Autodesk Inventor part; units mm, degrees
(part 2 of 2)
sketch "Sketch26" plane through (0, 0, 0) normal (0, -1, 0) x (1, 0, 0)
  circle A0 centre (0, 0) radius 23.8125 construction
  spline S0 degree 2 poles (-24.8851, 3.9966) (-24.5644, 3.9692) (-24.1006, 3.6837) (-23.9576, 3.4678) knots 0 0 0 1 2 2 2
  spline S1 degree 2 poles (-23.9576, 3.4678) (-23.7867, 3.2073) (-23.6758, 2.6148) (-23.7143, 2.1651) knots 0 0 0 1 2 2 2
  line L0 (-23.7143, 2.1651) -> (-23.8613, 0.4463)
  line L1 (-23.8613, 0.4463) -> (-28.1636, 0.8142)
  line L2 (-28.1636, 0.8142) -> (-28.0338, 2.3308)
  spline S2 degree 2 poles (-28.0338, 2.3308) (-27.9933, 2.805) (-27.8783, 3.2868) (-27.7451, 3.4897) knots 0 0 0 1 2 2 2
  spline S3 degree 2 poles (-27.7451, 3.4897) (-27.6031, 3.7128) (-27.1653, 3.9037) (-26.8934, 3.8804) knots 0 0 0 1 2 2 2
  spline S4 degree 2 poles (-26.8934, 3.8804) (-26.5796, 3.8536) (-26.1149, 3.4977) (-26.0237, 3.209) knots 0 0 0 1 2 2 2
  line L3 (-26.0237, 3.209) -> (-26.0027, 3.2072)
  spline S5 degree 2 poles (-26.0027, 3.2072) (-25.8848, 3.601) (-25.3244, 4.0342) (-24.8851, 3.9966) knots 0 0 0 1 2 2 2
  spline S6 degree 2 poles (-24.998, 2.8825) (-25.2002, 2.8997) (-25.4405, 2.7588) (-25.5135, 2.6034) knots 0 0 0 1 2 2 2
  spline S7 degree 2 poles (-25.5135, 2.6034) (-25.5602, 2.5091) (-25.5967, 2.1645) (-25.6212, 1.8786) knots 0 0 0 1 2 2 2
  line L4 (-25.6212, 1.8786) -> (-25.6382, 1.6799)
  line L5 (-25.6382, 1.6799) -> (-24.5539, 1.5872)
  line L6 (-24.5539, 1.5872) -> (-24.5488, 1.6465)
  spline S8 degree 2 poles (-24.5488, 1.6465) (-24.513, 2.0648) (-24.4961, 2.3865) (-24.555, 2.5601) knots 0 0 0 1 2 2 2
  spline S9 degree 2 poles (-24.555, 2.5601) (-24.6087, 2.7122) (-24.8411, 2.869) (-24.998, 2.8825) knots 0 0 0 1 2 2 2
  spline S10 degree 2 poles (-26.7746, 2.764) (-26.8792, 2.7729) (-27.1081, 2.6836) (-27.1665, 2.5762) knots 0 0 0 1 2 2 2
  spline S11 degree 2 poles (-27.1665, 2.5762) (-27.2242, 2.4758) (-27.2563, 2.1835) (-27.281, 1.8942) knots 0 0 0 1 2 2 2
  line L7 (-27.281, 1.8942) -> (-27.2873, 1.821)
  line L8 (-27.2873, 1.821) -> (-26.3738, 1.7428)
  line L9 (-26.3738, 1.7428) -> (-26.3622, 1.8788)
  spline S12 degree 2 poles (-26.3622, 1.8788) (-26.3386, 2.1542) (-26.33, 2.3783) (-26.3756, 2.5016) knots 0 0 0 1 2 2 2
  spline S13 degree 2 poles (-26.3756, 2.5016) (-26.4274, 2.6359) (-26.6317, 2.7518) (-26.7746, 2.764) knots 0 0 0 1 2 2 2
  spline S14 degree 2 poles (-24.2532, 7.8601) (-23.4729, 7.663) (-22.7924, 6.5852) (-22.9886, 5.8083) knots 0 0 0 1 2 2 2
  spline S15 degree 2 poles (-22.9886, 5.8083) (-23.184, 5.0348) (-24.2964, 4.4027) (-25.0768, 4.5998) knots 0 0 0 1 2 2 2
  spline S16 degree 2 poles (-25.0768, 4.5998) (-25.8638, 4.7986) (-26.5393, 5.8823) (-26.3439, 6.6558) knots 0 0 0 1 2 2 2
  spline S17 degree 2 poles (-26.3439, 6.6558) (-26.1486, 7.4293) (-25.0369, 8.0581) (-24.2532, 7.8601) knots 0 0 0 1 2 2 2
  spline S18 degree 2 poles (-24.501, 6.8508) (-24.7826, 6.9219) (-25.1823, 6.9254) (-25.3148, 6.8723) knots 0 0 0 1 2 2 2
  spline S19 degree 2 poles (-25.3148, 6.8723) (-25.4558, 6.8141) (-25.6031, 6.6167) (-25.6383, 6.4776) knots 0 0 0 1 2 2 2
  spline S20 degree 2 poles (-25.6383, 6.4776) (-25.6725, 6.3419) (-25.6451, 6.1076) (-25.552, 5.9902) knots 0 0 0 1 2 2 2
  spline S21 degree 2 poles (-25.552, 5.9902) (-25.4649, 5.878) (-25.1072, 5.6794) (-24.8155, 5.6057) knots 0 0 0 1 2 2 2
  spline S22 degree 2 poles (-24.8155, 5.6057) (-24.5271, 5.5328) (-24.1469, 5.5379) (-24.0186, 5.5885) knots 0 0 0 1 2 2 2
  spline S23 degree 2 poles (-24.0186, 5.5885) (-23.8903, 5.6391) (-23.7286, 5.8509) (-23.6926, 5.9933) knots 0 0 0 1 2 2 2
  spline S24 degree 2 poles (-23.6926, 5.9933) (-23.6626, 6.1121) (-23.7027, 6.3821) (-23.7856, 6.4824) knots 0 0 0 1 2 2 2
  spline S25 degree 2 poles (-23.7856, 6.4824) (-23.8829, 6.5972) (-24.2024, 6.7754) (-24.501, 6.8508) knots 0 0 0 1 2 2 2
  spline S26 degree 2 poles (-21.9439, 9.0922) (-22.1712, 8.5161) (-22.8546, 8.1763) (-23.3949, 8.3896) knots 0 0 0 1 2 2 2
  line L10 (-23.3949, 8.3896) -> (-24.8107, 8.9484)
  line L11 (-24.8107, 8.9484) -> (-24.9533, 8.5872)
  line L12 (-24.9533, 8.5872) -> (-25.6108, 8.8467)
  line L13 (-25.6108, 8.8467) -> (-25.4682, 9.208)
  line L14 (-25.4682, 9.208) -> (-26.334, 9.5497)
  line L15 (-26.334, 9.5497) -> (-25.9614, 10.4936)
  line L16 (-25.9614, 10.4936) -> (-25.0956, 10.1519)
  line L17 (-25.0956, 10.1519) -> (-24.7359, 11.0632)
  line L18 (-24.7359, 11.0632) -> (-24.0784, 10.8037)
  line L19 (-24.0784, 10.8037) -> (-24.4382, 9.8923)
  line L20 (-24.4382, 9.8923) -> (-23.3608, 9.4671)
  spline S27 degree 2 poles (-23.3608, 9.4671) (-23.2013, 9.4042) (-22.9611, 9.3169) (-22.8513, 9.3187) knots 0 0 0 1 2 2 2
  spline S28 degree 2 poles (-22.8513, 9.3187) (-22.7415, 9.3205) (-22.5551, 9.4688) (-22.4831, 9.6511) knots 0 0 0 1 2 2 2
  spline S29 degree 2 poles (-22.4831, 9.6511) (-22.4523, 9.7292) (-22.421, 9.999) (-22.4278, 10.0581) knots 0 0 0 1 2 2 2
  line L21 (-22.4278, 10.0581) -> (-22.3957, 10.1395)
  line L22 (-22.3957, 10.1395) -> (-21.7317, 9.8774)
  spline S30 degree 2 poles (-21.7317, 9.8774) (-21.753, 9.709) (-21.8436, 9.346) (-21.9439, 9.0922) knots 0 0 0 1 2 2 2
  spline S31 degree 2 poles (-20.887, 11.3108) (-21.1727, 10.7612) (-21.8875, 10.4939) (-22.4028, 10.7619) knots 0 0 0 1 2 2 2
  line L23 (-22.4028, 10.7619) -> (-23.7534, 11.464)
  line L24 (-23.7534, 11.464) -> (-23.9325, 11.1194)
  line L25 (-23.9325, 11.1194) -> (-24.5597, 11.4455)
  line L26 (-24.5597, 11.4455) -> (-24.3805, 11.7901)
  line L27 (-24.3805, 11.7901) -> (-25.2064, 12.2194)
  line L28 (-25.2064, 12.2194) -> (-24.7383, 13.1198)
  line L29 (-24.7383, 13.1198) -> (-23.9124, 12.6904)
  line L30 (-23.9124, 12.6904) -> (-23.4605, 13.5597)
  line L31 (-23.4605, 13.5597) -> (-22.8333, 13.2337)
  line L32 (-22.8333, 13.2337) -> (-23.2853, 12.3644)
  line L33 (-23.2853, 12.3644) -> (-22.2576, 11.8301)
  spline S32 degree 2 poles (-22.2576, 11.8301) (-22.1055, 11.751) (-21.8756, 11.6394) (-21.7662, 11.6298) knots 0 0 0 1 2 2 2
  spline S33 degree 2 poles (-21.7662, 11.6298) (-21.6568, 11.6203) (-21.456, 11.7486) (-21.3656, 11.9224) knots 0 0 0 1 2 2 2
  spline S34 degree 2 poles (-21.3656, 11.9224) (-21.3269, 11.9969) (-21.2679, 12.2621) (-21.2686, 12.3216) knots 0 0 0 1 2 2 2
  line L34 (-21.2686, 12.3216) -> (-21.2282, 12.3992)
  line L35 (-21.2282, 12.3992) -> (-20.5949, 12.0699)
  spline S35 degree 2 poles (-20.5949, 12.0699) (-20.6335, 11.9046) (-20.7611, 11.5529) (-20.887, 11.3108) knots 0 0 0 1 2 2 2
  spline S36 degree 2 poles (-19.9207, 15.9113) (-19.2601, 15.4515) (-19.0035, 14.203) (-19.4612, 13.5452) knots 0 0 0 1 2 2 2
  spline S37 degree 2 poles (-19.4612, 13.5452) (-19.9169, 12.8904) (-21.1809, 12.6914) (-21.8415, 13.1511) knots 0 0 0 1 2 2 2
  spline S38 degree 2 poles (-21.8415, 13.1511) (-22.5078, 13.6148) (-22.7575, 14.8671) (-22.3018, 15.522) knots 0 0 0 1 2 2 2
  spline S39 degree 2 poles (-22.3018, 15.522) (-21.8461, 16.1769) (-20.5841, 16.373) (-19.9207, 15.9113) knots 0 0 0 1 2 2 2
  spline S40 degree 2 poles (-20.5086, 15.0542) (-20.7469, 15.2201) (-21.1197, 15.3644) (-21.2625, 15.3615) knots 0 0 0 1 2 2 2
  spline S41 degree 2 poles (-21.2625, 15.3615) (-21.415, 15.3567) (-21.6224, 15.224) (-21.7044, 15.1063) knots 0 0 0 1 2 2 2
  spline S42 degree 2 poles (-21.7044, 15.1063) (-21.7843, 14.9914) (-21.8413, 14.7625) (-21.7956, 14.6198) knots 0 0 0 1 2 2 2
  spline S43 degree 2 poles (-21.7956, 14.6198) (-21.7537, 14.4841) (-21.4891, 14.172) (-21.2421, 14.0001) knots 0 0 0 1 2 2 2
  spline S44 degree 2 poles (-21.2421, 14.0001) (-20.998, 13.8302) (-20.6404, 13.7008) (-20.5025, 13.7029) knots 0 0 0 1 2 2 2
  spline S45 degree 2 poles (-20.5025, 13.7029) (-20.3647, 13.705) (-20.1386, 13.8461) (-20.0546, 13.9667) knots 0 0 0 1 2 2 2
  spline S46 degree 2 poles (-20.0546, 13.9667) (-19.9847, 14.0672) (-19.9269, 14.334) (-19.9691, 14.4572) knots 0 0 0 1 2 2 2
  spline S47 degree 2 poles (-19.9691, 14.4572) (-20.0197, 14.5989) (-20.2558, 14.8783) (-20.5086, 15.0542) knots 0 0 0 1 2 2 2
  line L36 (-15.498, 18.1366) -> (-16.628, 19.3073)
  spline S48 degree 2 poles (-16.628, 19.3073) (-16.7957, 19.481) (-17.0367, 19.7055) (-17.1399, 19.7519) knots 0 0 0 1 2 2 2
  spline S49 degree 2 poles (-17.1399, 19.7519) (-17.2455, 19.7958) (-17.442, 19.7374) (-17.5604, 19.6232) knots 0 0 0 1 2 2 2
  spline S50 degree 2 poles (-17.5604, 19.6232) (-17.6434, 19.543) (-17.7341, 19.3145) (-17.7641, 19.1541) knots 0 0 0 1 2 2 2
  line L37 (-17.7641, 19.1541) -> (-16.1627, 17.495)
  line L38 (-16.1627, 17.495) -> (-16.8978, 16.7854)
  line L39 (-16.8978, 16.7854) -> (-18.0278, 17.9561)
  spline S51 degree 2 poles (-18.0278, 17.9561) (-18.1931, 18.1273) (-18.4391, 18.3519) (-18.5422, 18.3983) knots 0 0 0 1 2 2 2
  spline S52 degree 2 poles (-18.5422, 18.3983) (-18.6478, 18.4422) (-18.8444, 18.3838) (-18.9627, 18.2696) knots 0 0 0 1 2 2 2
  spline S53 degree 2 poles (-18.9627, 18.2696) (-19.0508, 18.1845) (-19.1443, 17.9338) (-19.169, 17.7981) knots 0 0 0 1 2 2 2
  line L40 (-19.169, 17.7981) -> (-17.5675, 16.139)
  line L41 (-17.5675, 16.139) -> (-18.2976, 15.4342)
  line L42 (-18.2976, 15.4342) -> (-20.5601, 17.7781)
  line L43 (-20.5601, 17.7781) -> (-19.83, 18.4829)
  line L44 (-19.83, 18.4829) -> (-19.5797, 18.2236)
  spline S54 degree 2 poles (-19.5797, 18.2236) (-19.5468, 18.5472) (-19.3923, 19.027) (-19.1934, 19.219) knots 0 0 0 1 2 2 2
  spline S55 degree 2 poles (-19.1934, 19.219) (-18.9794, 19.4256) (-18.4552, 19.5376) (-18.1728, 19.4163) knots 0 0 0 1 2 2 2
  spline S56 degree 2 poles (-18.1728, 19.4163) (-18.1534, 19.8143) (-17.9849, 20.3855) (-17.7936, 20.5702) knots 0 0 0 1 2 2 2
  spline S57 degree 2 poles (-17.7936, 20.5702) (-17.6299, 20.7281) (-17.271, 20.8752) (-17.0808, 20.8545) knots 0 0 0 1 2 2 2
  spline S58 degree 2 poles (-17.0808, 20.8545) (-16.8732, 20.836) (-16.4761, 20.6211) (-16.2355, 20.3719) knots 0 0 0 1 2 2 2
  line L45 (-16.2355, 20.3719) -> (-14.7628, 18.8462)
  line L46 (-14.7628, 18.8462) -> (-15.498, 18.1366)
  line L47 (-9.4111, 21.9496) -> (-10.3726, 21.4473)
  line L48 (-10.3726, 21.4473) -> (-11.2588, 23.1438)
  line L49 (-11.2588, 23.1438) -> (-12.5646, 22.4617)
  line L50 (-12.5646, 22.4617) -> (-11.6783, 20.7652)
  line L51 (-11.6783, 20.7652) -> (-12.6398, 20.263)
  line L52 (-12.6398, 20.263) -> (-14.6391, 24.0902)
  line L53 (-14.6391, 24.0902) -> (-13.6776, 24.5925)
  line L54 (-13.6776, 24.5925) -> (-12.9453, 23.1906)
  line L55 (-12.9453, 23.1906) -> (-11.6396, 23.8727)
  line L56 (-11.6396, 23.8727) -> (-12.3719, 25.2746)
  line L57 (-12.3719, 25.2746) -> (-11.4104, 25.7768)
  line L58 (-11.4104, 25.7768) -> (-9.4111, 21.9496)
  spline S59 degree 2 poles (-7.0133, 22.6666) (-7.8923, 22.3827) (-9.0991, 22.9195) (-9.3497, 23.6954) knots 0 0 0 1 2 2 2
  spline S60 degree 2 poles (-9.3497, 23.6954) (-9.5949, 24.4546) (-9.0151, 25.6421) (-8.2293, 25.8959) knots 0 0 0 1 2 2 2
  spline S61 degree 2 poles (-8.2293, 25.8959) (-7.52, 26.125) (-6.5523, 25.5882) (-6.3221, 24.8756) knots 0 0 0 1 2 2 2
  line L59 (-6.3221, 24.8756) -> (-6.2092, 24.526)
  line L60 (-6.2092, 24.526) -> (-8.3303, 23.8408)
  spline S62 degree 2 poles (-8.3303, 23.8408) (-8.247, 23.6287) (-7.998, 23.3929) (-7.8435, 23.3472) knots 0 0 0 1 2 2 2
  spline S63 degree 2 poles (-7.8435, 23.3472) (-7.6924, 23.3004) (-7.3357, 23.3347) (-7.1393, 23.3982) knots 0 0 0 1 2 2 2
  spline S64 degree 2 poles (-7.1393, 23.3982) (-6.9728, 23.452) (-6.6701, 23.6306) (-6.554, 23.738) knots 0 0 0 1 2 2 2
  spline S65 degree 2 poles (-6.554, 23.738) (-6.4503, 23.8267) (-6.2903, 24.0144) (-6.2421, 24.0814) knots 0 0 0 1 2 2 2
  line L61 (-6.2421, 24.0814) -> (-6.1389, 24.1148)
  line L62 (-6.1389, 24.1148) -> (-5.8807, 23.3156)
  spline S66 degree 2 poles (-5.8807, 23.3156) (-5.9855, 23.2303) (-6.1529, 23.088) (-6.3131, 22.9921) knots 0 0 0 1 2 2 2
  spline S67 degree 2 poles (-6.3131, 22.9921) (-6.4556, 22.8983) (-6.7735, 22.7441) (-7.0133, 22.6666) knots 0 0 0 1 2 2 2
  spline S68 degree 2 poles (-7.3498, 24.8011) (-7.4554, 25.1053) (-7.8294, 25.3411) (-8.1058, 25.2518) knots 0 0 0 1 2 2 2
  spline S69 degree 2 poles (-8.1058, 25.2518) (-8.3888, 25.1604) (-8.5988, 24.7175) (-8.5218, 24.4224) knots 0 0 0 1 2 2 2
  line L63 (-8.5218, 24.4224) -> (-7.3498, 24.8011)
  line L64 (-2.0894, 23.7885) -> (-3.2634, 23.5956)
  line L65 (-3.2634, 23.5956) -> (-4.026, 24.4171)
  line L66 (-4.026, 24.4171) -> (-4.5029, 23.3919)
  line L67 (-4.5029, 23.3919) -> (-5.6528, 23.203)
  line L68 (-5.6528, 23.203) -> (-4.7328, 25.0066)
  line L69 (-4.7328, 25.0066) -> (-6.1602, 26.4211)
  line L70 (-6.1602, 26.4211) -> (-4.9862, 26.6139)
  line L71 (-4.9862, 26.6139) -> (-4.2368, 25.808)
  line L72 (-4.2368, 25.808) -> (-3.7812, 26.8119)
  line L73 (-3.7812, 26.8119) -> (-2.6314, 27.0009)
  line L74 (-2.6314, 27.0009) -> (-3.5352, 25.2282)
  line L75 (-3.5352, 25.2282) -> (-2.0894, 23.7885)
  line L76 (-0.4845, 23.8131) -> (-1.5088, 23.7701)
  line L77 (-1.5088, 23.7701) -> (-1.5566, 24.9099)
  line L78 (-1.5566, 24.9099) -> (-0.5323, 24.9529)
  line L79 (-0.5323, 24.9529) -> (-0.4845, 23.8131)
  line L80 (-0.5732, 25.9283) -> (-1.5976, 25.8853)
  line L81 (-1.5976, 25.8853) -> (-1.6454, 27.025)
  line L82 (-1.6454, 27.025) -> (-0.621, 27.068)
  line L83 (-0.621, 27.068) -> (-0.5732, 25.9283)
  spline S70 degree 2 poles (5.6673, 25.4002) (5.5806, 24.8471) (5.2742, 24.045) (5.0332, 23.7959) knots 0 0 0 1 2 2 2
  spline S71 degree 2 poles (5.0332, 23.7959) (4.7963, 23.5497) (4.1261, 23.3644) (3.6767, 23.4349) knots 0 0 0 1 2 2 2
  spline S72 degree 2 poles (3.6767, 23.4349) (3.2239, 23.5059) (2.6461, 23.8869) (2.4935, 24.2013) knots 0 0 0 1 2 2 2
  spline S73 degree 2 poles (2.4935, 24.2013) (2.3403, 24.5122) (2.2931, 25.3626) (2.3798, 25.9157) knots 0 0 0 1 2 2 2
  spline S74 degree 2 poles (2.3798, 25.9157) (2.4687, 26.4826) (2.7708, 27.257) (3.0168, 27.5159) knots 0 0 0 1 2 2 2
  spline S75 degree 2 poles (3.0168, 27.5159) (3.2618, 27.768) (3.9378, 27.9453) (4.3733, 27.877) knots 0 0 0 1 2 2 2
  spline S76 degree 2 poles (4.3733, 27.877) (4.8331, 27.8049) (5.4029, 27.418) (5.555, 27.1002) knots 0 0 0 1 2 2 2
  spline S77 degree 2 poles (5.555, 27.1002) (5.7046, 26.7898) (5.7514, 25.936) (5.6673, 25.4002) knots 0 0 0 1 2 2 2
  spline S78 degree 2 poles (4.5922, 25.5688) (4.7164, 26.3604) (4.5574, 27.0406) (4.2497, 27.0888) knots 0 0 0 1 2 2 2
  spline S79 degree 2 poles (4.2497, 27.0888) (3.9421, 27.1371) (3.579, 26.5388) (3.4544, 25.7437) knots 0 0 0 1 2 2 2
  spline S80 degree 2 poles (3.4544, 25.7437) (3.3318, 24.9624) (3.4927, 24.2713) (3.8003, 24.223) knots 0 0 0 1 2 2 2
  spline S81 degree 2 poles (3.8003, 24.223) (4.1045, 24.1753) (4.4692, 24.784) (4.5922, 25.5688) knots 0 0 0 1 2 2 2
  line L84 (6.9289, 22.7878) -> (5.9419, 23.065)
  line L85 (5.9419, 23.065) -> (6.2502, 24.1633)
  line L86 (6.2502, 24.1633) -> (7.2373, 23.8861)
  line L87 (7.2373, 23.8861) -> (6.9289, 22.7878)
  spline S82 degree 2 poles (11.1529, 22.7394) (11.0232, 22.4257) (10.5906, 21.9835) (10.3015, 21.8796) knots 0 0 0 1 2 2 2
  spline S83 degree 2 poles (10.3015, 21.8796) (10.0125, 21.7757) (9.35, 21.8034) (8.9296, 21.9771) knots 0 0 0 1 2 2 2
  spline S84 degree 2 poles (8.9296, 21.9771) (8.4846, 22.1648) (7.9045, 22.5749) (7.733, 22.7556) knots 0 0 0 1 2 2 2
  line L88 (7.733, 22.7556) -> (8.0925, 23.6255)
  line L89 (8.0925, 23.6255) -> (8.1831, 23.5881)
  spline S85 degree 2 poles (8.1831, 23.5881) (8.2433, 23.514) (8.3854, 23.3265) (8.5134, 23.2055) knots 0 0 0 1 2 2 2
  spline S86 degree 2 poles (8.5134, 23.2055) (8.6329, 23.0917) (8.8965, 22.8957) (9.0744, 22.8222) knots 0 0 0 1 2 2 2
  spline S87 degree 2 poles (9.0744, 22.8222) (9.2296, 22.758) (9.6239, 22.686) (9.7766, 22.744) knots 0 0 0 1 2 2 2
  spline S88 degree 2 poles (9.7766, 22.744) (9.8908, 22.7914) (10.0629, 22.9513) (10.1311, 23.1162) knots 0 0 0 1 2 2 2
  spline S89 degree 2 poles (10.1311, 23.1162) (10.1899, 23.2585) (10.1563, 23.5071) (10.0879, 23.6073) knots 0 0 0 1 2 2 2
  spline S90 degree 2 poles (10.0879, 23.6073) (9.9895, 23.754) (9.6229, 23.9661) (9.4838, 24.0236) knots 0 0 0 1 2 2 2
  spline S91 degree 2 poles (9.4838, 24.0236) (9.2639, 24.1145) (8.8173, 24.2157) (8.6493, 24.2398) knots 0 0 0 1 2 2 2
  line L90 (8.6493, 24.2398) -> (8.562, 24.2758)
  line L91 (8.562, 24.2758) -> (9.4882, 26.5169)
  line L92 (9.4882, 26.5169) -> (12.1335, 25.4236)
  line L93 (12.1335, 25.4236) -> (11.8221, 24.6701)
  line L94 (11.8221, 24.6701) -> (10.1243, 25.3718)
  line L95 (10.1243, 25.3718) -> (9.8503, 24.7089)
  spline S92 degree 2 poles (9.8503, 24.7089) (9.9338, 24.6819) (10.1597, 24.5962) (10.2211, 24.5708) knots 0 0 0 1 2 2 2
  spline S93 degree 2 poles (10.2211, 24.5708) (10.5089, 24.4518) (10.9459, 24.1349) (11.0872, 23.9364) knots 0 0 0 1 2 2 2
  spline S94 degree 2 poles (11.0872, 23.9364) (11.2521, 23.6941) (11.2999, 23.0951) (11.1529, 22.7394) knots 0 0 0 1 2 2 2
  line L96 (14.4928, 20.2273) -> (13.9948, 20.533)
  line L97 (13.9948, 20.533) -> (13.4622, 19.6651)
  line L98 (13.4622, 19.6651) -> (12.5705, 20.2123)
  line L99 (12.5705, 20.2123) -> (13.1031, 21.0802)
  line L100 (13.1031, 21.0802) -> (11.4807, 22.0759)
  line L101 (11.4807, 22.0759) -> (11.9016, 22.7618)
  line L102 (11.9016, 22.7618) -> (14.8047, 23.9198)
  line L103 (14.8047, 23.9198) -> (15.7262, 23.3543)
  line L104 (15.7262, 23.3543) -> (14.4011, 21.1951)
  line L105 (14.4011, 21.1951) -> (14.8992, 20.8894)
  line L106 (14.8992, 20.8894) -> (14.4928, 20.2273)
  line L107 (13.5094, 21.7423) -> (14.2781, 22.9949)
  line L108 (14.2781, 22.9949) -> (12.5759, 22.3152)
  line L109 (12.5759, 22.3152) -> (13.5094, 21.7423)
  spline S95 degree 2 poles (18.1713, 18.6304) (17.8068, 18.2054) (17.1246, 17.6842) (16.7886, 17.5989) knots 0 0 0 1 2 2 2
  spline S96 degree 2 poles (16.7886, 17.5989) (16.4577, 17.514) (15.7901, 17.7085) (15.4448, 18.0047) knots 0 0 0 1 2 2 2
  spline S97 degree 2 poles (15.4448, 18.0047) (15.0969, 18.3031) (14.8056, 18.9309) (14.841, 19.2786) knots 0 0 0 1 2 2 2
  spline S98 degree 2 poles (14.841, 19.2786) (14.8741, 19.6236) (15.2809, 20.3719) (15.6454, 20.7969) knots 0 0 0 1 2 2 2
  spline S99 degree 2 poles (15.6454, 20.7969) (16.019, 21.2325) (16.6829, 21.7325) (17.0283, 21.8235) knots 0 0 0 1 2 2 2
  spline S100 degree 2 poles (17.0283, 21.8235) (17.3692, 21.9091) (18.0375, 21.7047) (18.3722, 21.4177) knots 0 0 0 1 2 2 2
  spline S101 degree 2 poles (18.3722, 21.4177) (18.7254, 21.1147) (19.0068, 20.4861) (18.9692, 20.1358) knots 0 0 0 1 2 2 2
  spline S102 degree 2 poles (18.9692, 20.1358) (18.9334, 19.7931) (18.5244, 19.0421) (18.1713, 18.6304) knots 0 0 0 1 2 2 2
  spline S103 degree 2 poles (17.3452, 19.3389) (17.8669, 19.9471) (18.0892, 20.6094) (17.8528, 20.8121) knots 0 0 0 1 2 2 2
  spline S104 degree 2 poles (17.8528, 20.8121) (17.6164, 21.0149) (16.9931, 20.6966) (16.4691, 20.0857) knots 0 0 0 1 2 2 2
  spline S105 degree 2 poles (16.4691, 20.0857) (15.9543, 19.4855) (15.7278, 18.813) (15.9642, 18.6102) knots 0 0 0 1 2 2 2
  spline S106 degree 2 poles (15.9642, 18.6102) (16.198, 18.4098) (16.8281, 18.736) (17.3452, 19.3389) knots 0 0 0 1 2 2 2
  line L110 (19.6677, 13.4747) -> (18.2626, 15.3252)
  line L111 (18.2626, 15.3252) -> (18.8618, 15.7801)
  line L112 (18.8618, 15.7801) -> (19.2363, 15.2869)
  line L113 (19.2363, 15.2869) -> (21.477, 16.9881)
  line L114 (21.477, 16.9881) -> (21.1025, 17.4814)
  line L115 (21.1025, 17.4814) -> (21.7016, 17.9364)
  line L116 (21.7016, 17.9364) -> (23.1067, 16.0859)
  line L117 (23.1067, 16.0859) -> (22.5075, 15.6309)
  line L118 (22.5075, 15.6309) -> (22.133, 16.1242)
  line L119 (22.133, 16.1242) -> (19.8923, 14.4229)
  line L120 (19.8923, 14.4229) -> (20.2669, 13.9296)
  line L121 (20.2669, 13.9296) -> (19.6677, 13.4747)
  spline S107 degree 2 poles (23.8248, 10.5322) (23.2921, 10.2446) (22.2036, 10.2573) (21.7876, 10.49) knots 0 0 0 1 2 2 2
  spline S108 degree 2 poles (21.7876, 10.49) (21.4371, 10.6825) (20.9506, 11.3185) (20.7394, 11.7096) knots 0 0 0 1 2 2 2
  line L122 (20.7394, 11.7096) -> (20.0977, 12.8981)
  line L123 (20.0977, 12.8981) -> (23.8972, 14.9496)
  line L124 (23.8972, 14.9496) -> (24.5323, 13.7735)
  spline S109 degree 2 poles (24.5323, 13.7735) (24.7484, 13.3732) (25.0242, 12.6194) (24.9934, 12.2051) knots 0 0 0 1 2 2 2
  spline S110 degree 2 poles (24.9934, 12.2051) (24.9544, 11.7029) (24.3759, 10.8298) (23.8248, 10.5322) knots 0 0 0 1 2 2 2
  spline S111 degree 2 poles (23.3023, 11.5147) (23.6779, 11.7175) (24.074, 12.2654) (24.0819, 12.6117) knots 0 0 0 1 2 2 2
  spline S112 degree 2 poles (24.0819, 12.6117) (24.0818, 12.8622) (23.874, 13.2987) (23.7144, 13.5943) knots 0 0 0 1 2 2 2
  line L125 (23.7144, 13.5943) -> (23.7044, 13.6128)
  line L126 (23.7044, 13.6128) -> (21.3243, 12.3276)
  line L127 (21.3243, 12.3276) -> (21.3343, 12.3091)
  spline S113 degree 2 poles (21.3343, 12.3091) (21.5072, 11.9889) (21.7665, 11.5603) (22.0008, 11.4283) knots 0 0 0 1 2 2 2
  spline S114 degree 2 poles (22.0008, 11.4283) (22.2749, 11.2741) (22.9266, 11.3118) (23.3023, 11.5147) knots 0 0 0 1 2 2 2
  line L128 (24.4852, 8.5487) -> (24.1281, 9.5098)
  line L129 (24.1281, 9.5098) -> (25.1974, 9.9071)
  line L130 (25.1974, 9.9071) -> (25.5545, 8.946)
  line L131 (25.5545, 8.946) -> (24.4852, 8.5487)
  line L132 (22.5007, 7.8114) -> (22.1436, 8.7725)
  line L133 (22.1436, 8.7725) -> (23.2129, 9.1698)
  line L134 (23.2129, 9.1698) -> (23.57, 8.2087)
  line L135 (23.57, 8.2087) -> (22.5007, 7.8114)
  line L136 (23.7556, 2.2444) -> (23.3062, 5.0606)
  line L137 (23.3062, 5.0606) -> (24.0491, 5.1792)
  line L138 (24.0491, 5.1792) -> (24.1925, 4.2807)
  line L139 (24.1925, 4.2807) -> (26.4489, 4.6408)
  line L140 (26.4489, 4.6408) -> (26.3056, 5.5393)
  line L141 (26.3056, 5.5393) -> (27.0001, 5.6501)
  spline S115 degree 2 poles (27.0001, 5.6501) (27.0315, 5.4531) (27.1457, 5.0709) (27.2197, 4.9623) knots 0 0 0 1 2 2 2
  spline S116 degree 2 poles (27.2197, 4.9623) (27.3103, 4.8386) (27.5661, 4.7235) (27.7411, 4.7372) knots 0 0 0 1 2 2 2
  line L142 (27.7411, 4.7372) -> (27.89, 3.8042)
  line L143 (27.89, 3.8042) -> (24.3585, 3.2406)
  line L144 (24.3585, 3.2406) -> (24.4986, 2.363)
  line L145 (24.4986, 2.363) -> (23.7556, 2.2444)
  line L146 (23.8138, 0.4435) -> (23.7728, 1.468)
  line L147 (23.7728, 1.468) -> (24.9126, 1.5137)
  line L148 (24.9126, 1.5137) -> (24.9537, 0.4892)
  line L149 (24.9537, 0.4892) -> (23.8138, 0.4435)
  spline S117 degree 2 poles (25.0716, -3.5891) (24.7332, -3.5626) (24.1791, -3.2876) (23.991, -3.0447) knots 0 0 0 1 2 2 2
  spline S118 degree 2 poles (23.991, -3.0447) (23.8029, -2.8019) (23.6248, -2.1631) (23.6603, -1.7096) knots 0 0 0 1 2 2 2
  spline S119 degree 2 poles (23.6603, -1.7096) (23.7014, -1.2285) (23.9125, -0.5501) (24.0314, -0.3312) knots 0 0 0 1 2 2 2
  line L150 (24.0314, -0.3312) -> (24.9698, -0.4047)
  line L151 (24.9698, -0.4047) -> (24.9621, -0.5023)
  spline S120 degree 2 poles (24.9621, -0.5023) (24.9102, -0.5825) (24.7758, -0.7756) (24.7002, -0.9346) knots 0 0 0 1 2 2 2
  spline S121 degree 2 poles (24.7002, -0.9346) (24.6289, -1.0835) (24.5238, -1.3946) (24.5088, -1.5865) knots 0 0 0 1 2 2 2
  spline S122 degree 2 poles (24.5088, -1.5865) (24.4957, -1.754) (24.5488, -2.1512) (24.6511, -2.2786) knots 0 0 0 1 2 2 2
  spline S123 degree 2 poles (24.6511, -2.2786) (24.7315, -2.3726) (24.9367, -2.4869) (25.1146, -2.5009) knots 0 0 0 1 2 2 2
  spline S124 degree 2 poles (25.1146, -2.5009) (25.2681, -2.5129) (25.4942, -2.4042) (25.5684, -2.3082) knots 0 0 0 1 2 2 2
  spline S125 degree 2 poles (25.5684, -2.3082) (25.6776, -2.1694) (25.7661, -1.7551) (25.7779, -1.6051) knots 0 0 0 1 2 2 2
  spline S126 degree 2 poles (25.7779, -1.6051) (25.7964, -1.3679) (25.7549, -0.9119) (25.7259, -0.7446) knots 0 0 0 1 2 2 2
  line L152 (25.7259, -0.7446) -> (25.7333, -0.6504)
  line L153 (25.7333, -0.6504) -> (28.1508, -0.8397)
  line L154 (28.1508, -0.8397) -> (27.9275, -3.6933)
  line L155 (27.9275, -3.6933) -> (27.1146, -3.6296)
  line L156 (27.1146, -3.6296) -> (27.258, -1.7982)
  line L157 (27.258, -1.7982) -> (26.5428, -1.7422)
  spline S127 degree 2 poles (26.5428, -1.7422) (26.543, -1.83) (26.5311, -2.0712) (26.5259, -2.1375) knots 0 0 0 1 2 2 2
  spline S128 degree 2 poles (26.5259, -2.1375) (26.5016, -2.448) (26.3351, -2.9614) (26.1899, -3.1571) knots 0 0 0 1 2 2 2
  spline S129 degree 2 poles (26.1899, -3.1571) (26.0103, -3.3888) (25.4553, -3.6191) (25.0716, -3.5891) knots 0 0 0 1 2 2 2
  line L158 (27.4168, -7.1888) -> (25.7876, -6.6482)
  line L159 (25.7876, -6.6482) -> (25.9164, -6.0674)
  line L160 (25.9164, -6.0674) -> (27.6214, -6.2664)
  line L161 (27.6214, -6.2664) -> (27.4168, -7.1888)
  line L162 (27.6812, -5.9965) -> (26.052, -5.4559)
  line L163 (26.052, -5.4559) -> (26.1809, -4.8752)
  line L164 (26.1809, -4.8752) -> (27.8858, -5.0742)
  line L165 (27.8858, -5.0742) -> (27.6812, -5.9965)
  spline S130 degree 2 poles (22.5039, -13.1325) (21.5577, -12.6779) (20.9609, -11.1488) (21.3822, -10.272) knots 0 0 0 1 2 2 2
  spline S131 degree 2 poles (21.3822, -10.272) (21.805, -9.392) (23.3813, -8.9149) (24.3149, -9.3635) knots 0 0 0 1 2 2 2
  spline S132 degree 2 poles (24.3149, -9.3635) (25.2517, -9.8136) (25.861, -11.3409) (25.4382, -12.2209) knots 0 0 0 1 2 2 2
  spline S133 degree 2 poles (25.4382, -12.2209) (25.0169, -13.0977) (23.447, -13.5856) (22.5039, -13.1325) knots 0 0 0 1 2 2 2
  spline S134 degree 2 poles (22.9889, -12.1232) (23.339, -12.2915) (23.896, -12.3844) (24.1097, -12.3357) knots 0 0 0 1 2 2 2
  spline S135 degree 2 poles (24.1097, -12.3357) (24.3297, -12.29) (24.62, -12.0412) (24.7018, -11.8709) knots 0 0 0 1 2 2 2
  spline S136 degree 2 poles (24.7018, -11.8709) (24.7882, -11.6911) (24.7998, -11.3357) (24.701, -11.1213) knots 0 0 0 1 2 2 2
  spline S137 degree 2 poles (24.701, -11.1213) (24.6072, -10.9287) (24.1769, -10.5395) (23.83, -10.3728) knots 0 0 0 1 2 2 2
  spline S138 degree 2 poles (23.83, -10.3728) (23.4704, -10.2) (22.9291, -10.1146) (22.7092, -10.1603) knots 0 0 0 1 2 2 2
  spline S139 degree 2 poles (22.7092, -10.1603) (22.4892, -10.206) (22.1974, -10.4579) (22.1155, -10.6282) knots 0 0 0 1 2 2 2
  spline S140 degree 2 poles (22.1155, -10.6282) (22.0322, -10.8017) (22.0258, -11.1946) (22.1275, -11.3871) knots 0 0 0 1 2 2 2
  spline S141 degree 2 poles (22.1275, -11.3871) (22.2372, -11.5951) (22.623, -11.9474) (22.9889, -12.1232) knots 0 0 0 1 2 2 2
  spline S142 degree 2 poles (19.6411, -17.1107) (19.1547, -16.7503) (18.7047, -15.7591) (18.739, -15.2837) knots 0 0 0 1 2 2 2
  spline S143 degree 2 poles (18.739, -15.2837) (18.7648, -14.8846) (19.1344, -14.1742) (19.399, -13.8172) knots 0 0 0 1 2 2 2
  line L166 (19.399, -13.8172) -> (20.2032, -12.7321)
  line L167 (20.2032, -12.7321) -> (23.6724, -15.3031)
  line L168 (23.6724, -15.3031) -> (22.8765, -16.377)
  spline S144 degree 2 poles (22.8765, -16.377) (22.6056, -16.7425) (22.0399, -17.3119) (21.6516, -17.4597) knots 0 0 0 1 2 2 2
  spline S145 degree 2 poles (21.6516, -17.4597) (21.1803, -17.6373) (20.1443, -17.4837) (19.6411, -17.1107) knots 0 0 0 1 2 2 2
  spline S146 degree 2 poles (20.3093, -16.2209) (20.6522, -16.4751) (21.3164, -16.6015) (21.6333, -16.4618) knots 0 0 0 1 2 2 2
  spline S147 degree 2 poles (21.6333, -16.4618) (21.8602, -16.3555) (22.1674, -15.9821) (22.3674, -15.7122) knots 0 0 0 1 2 2 2
  line L169 (22.3674, -15.7122) -> (22.3799, -15.6954)
  line L170 (22.3799, -15.6954) -> (20.2068, -14.0848)
  line L171 (20.2068, -14.0848) -> (20.1943, -14.1017)
  spline S148 degree 2 poles (20.1943, -14.1017) (19.9776, -14.3941) (19.6993, -14.8107) (19.6792, -15.0788) knots 0 0 0 1 2 2 2
  spline S149 degree 2 poles (19.6792, -15.0788) (19.6558, -15.3925) (19.9663, -15.9667) (20.3093, -16.2209) knots 0 0 0 1 2 2 2
  line L172 (18.1248, -18.5499) -> (18.8437, -17.8189)
  line L173 (18.8437, -17.8189) -> (19.657, -18.6189)
  line L174 (19.657, -18.6189) -> (18.938, -19.3498)
  line L175 (18.938, -19.3498) -> (18.1248, -18.5499)
  line L176 (16.6155, -17.0653) -> (17.3345, -16.3344)
  line L177 (17.3345, -16.3344) -> (18.1477, -17.1343)
  line L178 (18.1477, -17.1343) -> (17.4288, -17.8652)
  line L179 (17.4288, -17.8652) -> (16.6155, -17.0653)
  line L180 (11.9467, -20.6705) -> (14.573, -18.8885)
  line L181 (14.573, -18.8885) -> (14.9679, -19.4706)
  spline S150 degree 2 poles (14.9679, -19.4706) (14.8156, -19.9629) (14.6011, -20.7935) (14.5448, -21.1404) knots 0 0 0 1 2 2 2
  spline S151 degree 2 poles (14.5448, -21.1404) (14.4679, -21.5943) (14.5182, -22.1733) (14.6676, -22.3933) knots 0 0 0 1 2 2 2
  spline S152 degree 2 poles (14.6676, -22.3933) (14.8365, -22.6424) (15.3155, -22.7064) (15.5819, -22.5256) knots 0 0 0 1 2 2 2
  spline S153 degree 2 poles (15.5819, -22.5256) (15.718, -22.4333) (15.916, -22.2017) (16.0052, -22.0651) knots 0 0 0 1 2 2 2
  spline S154 degree 2 poles (16.0052, -22.0651) (16.0895, -21.9275) (16.1846, -21.6938) (16.2084, -21.6354) knots 0 0 0 1 2 2 2
  line L182 (16.2084, -21.6354) -> (16.2779, -21.5883)
  line L183 (16.2779, -21.5883) -> (16.8064, -22.3672)
  spline S155 degree 2 poles (16.8064, -22.3672) (16.7049, -22.5417) (16.1643, -23.1284) (15.866, -23.3308) knots 0 0 0 1 2 2 2
  spline S156 degree 2 poles (15.866, -23.3308) (15.229, -23.763) (14.1895, -23.6395) (13.8418, -23.127) knots 0 0 0 1 2 2 2
  spline S157 degree 2 poles (13.8418, -23.127) (13.6276, -22.8114) (13.5133, -22.0009) (13.6221, -21.4197) knots 0 0 0 1 2 2 2
  spline S158 degree 2 poles (13.6221, -21.4197) (13.6939, -21.0581) (13.8762, -20.448) (13.9189, -20.3176) knots 0 0 0 1 2 2 2
  line L184 (13.9189, -20.3176) -> (12.4045, -21.3452)
  line L185 (12.4045, -21.3452) -> (11.9467, -20.6705)
  line L186 (10.4997, -21.3788) -> (11.41, -20.9072)
  line L187 (11.41, -20.9072) -> (11.9348, -21.9201)
  line L188 (11.9348, -21.9201) -> (11.0244, -22.3917)
  line L189 (11.0244, -22.3917) -> (10.4997, -21.3788)
  spline S159 degree 2 poles (7.3809, -24.2278) (7.2614, -23.9101) (7.2755, -23.2917) (7.4157, -23.0184) knots 0 0 0 1 2 2 2
  spline S160 degree 2 poles (7.4157, -23.0184) (7.5559, -22.7451) (8.0588, -22.3129) (8.4845, -22.1527) knots 0 0 0 1 2 2 2
  spline S161 degree 2 poles (8.4845, -22.1527) (8.9378, -21.986) (9.6417, -21.8894) (9.8903, -21.9043) knots 0 0 0 1 2 2 2
  line L190 (9.8903, -21.9043) -> (10.2217, -22.7853)
  line L191 (10.2217, -22.7853) -> (10.13, -22.8198)
  spline S162 degree 2 poles (10.13, -22.8198) (10.0354, -22.8068) (9.8035, -22.7669) (9.6274, -22.7659) knots 0 0 0 1 2 2 2
  spline S163 degree 2 poles (9.6274, -22.7659) (9.4624, -22.7644) (9.136, -22.8012) (8.9559, -22.869) knots 0 0 0 1 2 2 2
  spline S164 degree 2 poles (8.9559, -22.869) (8.7986, -22.9281) (8.4614, -23.1447) (8.3895, -23.2914) knots 0 0 0 1 2 2 2
  spline S165 degree 2 poles (8.3895, -23.2914) (8.3384, -23.404) (8.3218, -23.6383) (8.3847, -23.8054) knots 0 0 0 1 2 2 2
  spline S166 degree 2 poles (8.3847, -23.8054) (8.4389, -23.9495) (8.6332, -24.1082) (8.7516, -24.1347) knots 0 0 0 1 2 2 2
  spline S167 degree 2 poles (8.7516, -24.1347) (8.9236, -24.1746) (9.3363, -24.0792) (9.4772, -24.0262) knots 0 0 0 1 2 2 2
  spline S168 degree 2 poles (9.4772, -24.0262) (9.6999, -23.9424) (10.0953, -23.7115) (10.2344, -23.6143) knots 0 0 0 1 2 2 2
  line L192 (10.2344, -23.6143) -> (10.3228, -23.581)
  line L193 (10.3228, -23.581) -> (11.1766, -25.8507)
  line L194 (11.1766, -25.8507) -> (8.4976, -26.8584)
  line L195 (8.4976, -26.8584) -> (8.2105, -26.0953)
  line L196 (8.2105, -26.0953) -> (9.9299, -25.4485)
  line L197 (9.9299, -25.4485) -> (9.6774, -24.7771)
  spline S169 degree 2 poles (9.6774, -24.7771) (9.598, -24.8145) (9.3745, -24.906) (9.3122, -24.9294) knots 0 0 0 1 2 2 2
  spline S170 degree 2 poles (9.3122, -24.9294) (9.0207, -25.0391) (8.4851, -25.106) (8.2463, -25.0575) knots 0 0 0 1 2 2 2
  spline S171 degree 2 poles (8.2463, -25.0575) (7.9604, -24.9931) (7.5164, -24.5881) (7.3809, -24.2278) knots 0 0 0 1 2 2 2
  line L198 (6.3072, -27.6121) -> (6.1059, -25.9074)
  line L199 (6.1059, -25.9074) -> (6.6865, -25.7778)
  line L200 (6.6865, -25.7778) -> (7.2293, -27.4063)
  line L201 (7.2293, -27.4063) -> (6.3072, -27.6121)
  line L202 (5.1153, -27.8782) -> (4.9141, -26.1735)
  line L203 (4.9141, -26.1735) -> (5.4946, -26.0439)
  line L204 (5.4946, -26.0439) -> (6.0374, -27.6723)
  line L205 (6.0374, -27.6723) -> (5.1153, -27.8782)
  line L206 (-2.0425, -23.7946) -> (-0.9578, -23.8046)
  line L207 (-0.9578, -23.8046) -> (-0.9755, -25.7186)
  line L208 (-0.9755, -25.7186) -> (0.4976, -25.7323)
  line L209 (0.4976, -25.7323) -> (0.5153, -23.8183)
  line L210 (0.5153, -23.8183) -> (1.6, -23.8284)
  line L211 (1.6, -23.8284) -> (1.5599, -28.1462)
  line L212 (1.5599, -28.1462) -> (0.4752, -28.1361)
  line L213 (0.4752, -28.1361) -> (0.4899, -26.5546)
  line L214 (0.4899, -26.5546) -> (-0.9832, -26.5409)
  line L215 (-0.9832, -26.5409) -> (-0.9979, -28.1224)
  line L216 (-0.9979, -28.1224) -> (-2.0826, -28.1124)
  line L217 (-2.0826, -28.1124) -> (-2.0425, -23.7946)
  spline S172 degree 2 poles (-4.0869, -23.3987) (-3.4751, -23.4949) (-2.9945, -24.0877) (-3.0848, -24.6615) knots 0 0 0 1 2 2 2
  line L218 (-3.0848, -24.6615) -> (-3.3213, -26.1652)
  line L219 (-3.3213, -26.1652) -> (-2.9376, -26.2255)
  line L220 (-2.9376, -26.2255) -> (-3.0475, -26.9238)
  line L221 (-3.0475, -26.9238) -> (-3.4312, -26.8634)
  line L222 (-3.4312, -26.8634) -> (-3.5759, -27.7829)
  line L223 (-3.5759, -27.7829) -> (-4.5783, -27.6252)
  line L224 (-4.5783, -27.6252) -> (-4.4336, -26.7057)
  line L225 (-4.4336, -26.7057) -> (-5.4015, -26.5534)
  line L226 (-5.4015, -26.5534) -> (-5.2916, -25.8552)
  line L227 (-5.2916, -25.8552) -> (-4.3238, -26.0074)
  line L228 (-4.3238, -26.0074) -> (-4.1438, -24.8633)
  spline S173 degree 2 poles (-4.1438, -24.8633) (-4.1171, -24.6939) (-4.0843, -24.4405) (-4.11, -24.3337) knots 0 0 0 1 2 2 2
  spline S174 degree 2 poles (-4.11, -24.3337) (-4.1357, -24.2269) (-4.3212, -24.0773) (-4.5148, -24.0469) knots 0 0 0 1 2 2 2
  spline S175 degree 2 poles (-4.5148, -24.0469) (-4.5977, -24.0338) (-4.8679, -24.0622) (-4.9241, -24.0817) knots 0 0 0 1 2 2 2
  line L229 (-4.9241, -24.0817) -> (-5.0105, -24.0681)
  line L230 (-5.0105, -24.0681) -> (-4.8995, -23.3629)
  spline S176 degree 2 poles (-4.8995, -23.3629) (-4.7305, -23.347) (-4.3565, -23.3562) (-4.0869, -23.3987) knots 0 0 0 1 2 2 2
  line L231 (-6.9892, -24.9751) -> (-5.9966, -25.2317)
  line L232 (-5.9966, -25.2317) -> (-6.2822, -26.3362)
  line L233 (-6.2822, -26.3362) -> (-7.2748, -26.0795)
  line L234 (-7.2748, -26.0795) -> (-6.9892, -24.9751)
  line L235 (-6.4593, -22.9255) -> (-5.4666, -23.1821)
  line L236 (-5.4666, -23.1821) -> (-5.7522, -24.2866)
  line L237 (-5.7522, -24.2866) -> (-6.7448, -24.0299)
  line L238 (-6.7448, -24.0299) -> (-6.4593, -22.9255)
  spline S177 degree 2 poles (-12.3892, -21.913) (-12.2506, -21.6263) (-11.8125, -21.259) (-11.5285, -21.1943) knots 0 0 0 1 2 2 2
  spline S178 degree 2 poles (-11.5285, -21.1943) (-11.2445, -21.1295) (-10.6017, -21.2228) (-10.2016, -21.4163) knots 0 0 0 1 2 2 2
  spline S179 degree 2 poles (-10.2016, -21.4163) (-9.748, -21.6357) (-9.1722, -22.1008) (-9.0132, -22.2943) knots 0 0 0 1 2 2 2
  line L239 (-9.0132, -22.2943) -> (-9.4215, -23.1385)
  line L240 (-9.4215, -23.1385) -> (-9.516, -23.0928)
  spline S180 degree 2 poles (-9.516, -23.0928) (-9.6647, -22.8538) (-10.1436, -22.3733) (-10.383, -22.2575) knots 0 0 0 1 2 2 2
  spline S181 degree 2 poles (-10.383, -22.2575) (-10.5248, -22.189) (-10.8799, -22.0794) (-11.033, -22.1064) knots 0 0 0 1 2 2 2
  spline S182 degree 2 poles (-11.033, -22.1064) (-11.1531, -22.1299) (-11.3532, -22.2703) (-11.437, -22.4435) knots 0 0 0 1 2 2 2
  spline S183 degree 2 poles (-11.437, -22.4435) (-11.5208, -22.6168) (-11.4595, -22.8758) (-11.3548, -22.9808) knots 0 0 0 1 2 2 2
  spline S184 degree 2 poles (-11.3548, -22.9808) (-11.2502, -23.0859) (-10.9051, -23.2644) (-10.7696, -23.33) knots 0 0 0 1 2 2 2
  line L241 (-10.7696, -23.33) -> (-10.6027, -23.4107)
  line L242 (-10.6027, -23.4107) -> (-10.9333, -24.0943)
  line L243 (-10.9333, -24.0943) -> (-11.0877, -24.0196)
  spline S185 degree 2 poles (-11.0877, -24.0196) (-11.2641, -23.9343) (-11.5785, -23.821) (-11.7054, -23.818) knots 0 0 0 1 2 2 2
  spline S186 degree 2 poles (-11.7054, -23.818) (-11.8337, -23.8181) (-12.0356, -23.9382) (-12.1087, -24.0894) knots 0 0 0 1 2 2 2
  spline S187 degree 2 poles (-12.1087, -24.0894) (-12.1666, -24.2091) (-12.128, -24.4104) (-12.069, -24.4895) knots 0 0 0 1 2 2 2
  spline S188 degree 2 poles (-12.069, -24.4895) (-11.9974, -24.5824) (-11.7606, -24.7358) (-11.6724, -24.7785) knots 0 0 0 1 2 2 2
  spline S189 degree 2 poles (-11.6724, -24.7785) (-11.5306, -24.8471) (-11.1994, -24.9257) (-11.0349, -24.9391) knots 0 0 0 1 2 2 2
  spline S190 degree 2 poles (-11.0349, -24.9391) (-10.9048, -24.9515) (-10.6014, -24.935) (-10.528, -24.9278) knots 0 0 0 1 2 2 2
  line L244 (-10.528, -24.9278) -> (-10.4461, -24.9674)
  line L245 (-10.4461, -24.9674) -> (-10.8483, -25.799)
  spline S191 degree 2 poles (-10.8483, -25.799) (-11.0911, -25.7866) (-11.8492, -25.6181) (-12.2051, -25.4459) knots 0 0 0 1 2 2 2
  spline S192 degree 2 poles (-12.2051, -25.4459) (-12.5516, -25.2783) (-13.004, -24.9118) (-13.1272, -24.7084) knots 0 0 0 1 2 2 2
  spline S193 degree 2 poles (-13.1272, -24.7084) (-13.2663, -24.4895) (-13.2819, -24.0155) (-13.1676, -23.7793) knots 0 0 0 1 2 2 2
  spline S194 degree 2 poles (-13.1676, -23.7793) (-13.0061, -23.4454) (-12.381, -23.1336) (-12.031, -23.2135) knots 0 0 0 1 2 2 2
  line L246 (-12.031, -23.2135) -> (-12.0127, -23.1757)
  spline S195 degree 2 poles (-12.0127, -23.1757) (-12.1422, -23.0897) (-12.358, -22.861) (-12.4292, -22.6866) knots 0 0 0 1 2 2 2
  spline S196 degree 2 poles (-12.4292, -22.6866) (-12.497, -22.5294) (-12.4959, -22.1335) (-12.3892, -21.913) knots 0 0 0 1 2 2 2
  line L247 (-13.2544, -19.7893) -> (-12.3905, -20.3415)
  line L248 (-12.3905, -20.3415) -> (-13.0049, -21.3026)
  line L249 (-13.0049, -21.3026) -> (-13.8687, -20.7505)
  line L250 (-13.8687, -20.7505) -> (-13.2544, -19.7893)
  spline S197 degree 2 poles (-17.7558, -19.0268) (-17.4008, -18.5939) (-16.7303, -18.0577) (-16.3963, -17.965) knots 0 0 0 1 2 2 2
  spline S198 degree 2 poles (-16.3963, -17.965) (-16.0673, -17.8728) (-15.3956, -18.0526) (-15.0439, -18.341) knots 0 0 0 1 2 2 2
  spline S199 degree 2 poles (-15.0439, -18.341) (-14.6894, -18.6317) (-14.3843, -19.253) (-14.4121, -19.6013) knots 0 0 0 1 2 2 2
  spline S200 degree 2 poles (-14.4121, -19.6013) (-14.4376, -19.947) (-14.8277, -20.7041) (-15.1827, -21.137) knots 0 0 0 1 2 2 2
  spline S201 degree 2 poles (-15.1827, -21.137) (-15.5466, -21.5807) (-16.1994, -22.0953) (-16.5427, -22.1938) knots 0 0 0 1 2 2 2
  spline S202 degree 2 poles (-16.5427, -22.1938) (-16.8816, -22.287) (-17.5543, -22.0974) (-17.8952, -21.8178) knots 0 0 0 1 2 2 2
  spline S203 degree 2 poles (-17.8952, -21.8178) (-18.255, -21.5227) (-18.5503, -20.9004) (-18.5203, -20.5494) knots 0 0 0 1 2 2 2
  spline S204 degree 2 poles (-18.5203, -20.5494) (-18.4921, -20.206) (-18.0998, -19.4461) (-17.7558, -19.0268) knots 0 0 0 1 2 2 2
  spline S205 degree 2 poles (-16.9144, -19.7169) (-17.4225, -20.3365) (-17.6301, -21.0034) (-17.3893, -21.2009) knots 0 0 0 1 2 2 2
  spline S206 degree 2 poles (-17.3893, -21.2009) (-17.1485, -21.3984) (-16.5323, -21.0665) (-16.022, -20.4442) knots 0 0 0 1 2 2 2
  spline S207 degree 2 poles (-16.022, -20.4442) (-15.5205, -19.8327) (-15.309, -19.1554) (-15.5498, -18.9579) knots 0 0 0 1 2 2 2
  spline S208 degree 2 poles (-15.5498, -18.9579) (-15.7879, -18.7626) (-16.4107, -19.1027) (-16.9144, -19.7169) knots 0 0 0 1 2 2 2
  line L251 (-20.7491, -19.2791) -> (-19.374, -18.2517)
  line L252 (-19.374, -18.2517) -> (-18.9712, -18.6895)
  line L253 (-18.9712, -18.6895) -> (-20.1095, -19.9744)
  line L254 (-20.1095, -19.9744) -> (-20.7491, -19.2791)
  line L255 (-21.5759, -18.3804) -> (-20.2008, -17.353)
  line L256 (-20.2008, -17.353) -> (-19.798, -17.7908)
  line L257 (-19.798, -17.7908) -> (-20.9363, -19.0757)
  line L258 (-20.9363, -19.0757) -> (-21.5759, -18.3804)
  line L259 (-25.3583, -12.3409) -> (-20.8773, -11.4649)
  line L260 (-20.8773, -11.4649) -> (-20.3118, -12.4435)
  line L261 (-20.3118, -12.4435) -> (-23.308, -15.8886)
  line L262 (-23.308, -15.8886) -> (-23.87, -14.9161)
  line L263 (-23.87, -14.9161) -> (-21.8052, -12.6356)
  line L264 (-21.8052, -12.6356) -> (-24.8102, -13.2892)
  line L265 (-24.8102, -13.2892) -> (-25.3583, -12.3409)
  spline S209 degree 2 poles (-25.3864, -5.7289) (-24.8492, -5.571) (-23.9932, -5.5053) (-23.665, -5.6167) knots 0 0 0 1 2 2 2
  spline S210 degree 2 poles (-23.665, -5.6167) (-23.3412, -5.7258) (-22.8872, -6.2525) (-22.7589, -6.6889) knots 0 0 0 1 2 2 2
  spline S211 degree 2 poles (-22.7589, -6.6889) (-22.6296, -7.1287) (-22.7273, -7.8139) (-22.9463, -8.0862) knots 0 0 0 1 2 2 2
  spline S212 degree 2 poles (-22.9463, -8.0862) (-23.162, -8.3575) (-23.9106, -8.7636) (-24.4478, -8.9215) knots 0 0 0 1 2 2 2
  spline S213 degree 2 poles (-24.4478, -8.9215) (-24.9983, -9.0834) (-25.8275, -9.1411) (-26.1668, -9.0293) knots 0 0 0 1 2 2 2
  spline S214 degree 2 poles (-26.1668, -9.0293) (-26.4993, -8.9155) (-26.9485, -8.3801) (-27.0728, -7.9571) knots 0 0 0 1 2 2 2
  spline S215 degree 2 poles (-27.0728, -7.9571) (-27.2041, -7.5106) (-27.0978, -6.8302) (-26.8754, -6.5569) knots 0 0 0 1 2 2 2
  spline S216 degree 2 poles (-26.8754, -6.5569) (-26.6587, -6.289) (-25.9067, -5.8819) (-25.3864, -5.7289) knots 0 0 0 1 2 2 2
  spline S217 degree 2 poles (-25.0794, -6.773) (-25.8482, -6.999) (-26.3952, -7.4333) (-26.3074, -7.7321) knots 0 0 0 1 2 2 2
  spline S218 degree 2 poles (-26.3074, -7.7321) (-26.2196, -8.0309) (-25.5235, -8.1035) (-24.7514, -7.8765) knots 0 0 0 1 2 2 2
  spline S219 degree 2 poles (-24.7514, -7.8765) (-23.9926, -7.6534) (-23.4365, -7.2127) (-23.5244, -6.9139) knots 0 0 0 1 2 2 2
  spline S220 degree 2 poles (-23.5244, -6.9139) (-23.6112, -6.6185) (-24.3174, -6.5489) (-25.0794, -6.773) knots 0 0 0 1 2 2 2
  spline S221 degree 2 poles (-25.0272, -1.4828) (-24.753, -1.4476) (-24.2481, -1.6158) (-24.0466, -1.8122) knots 0 0 0 1 2 2 2
  spline S222 degree 2 poles (-24.0466, -1.8122) (-23.845, -2.0087) (-23.5702, -2.612) (-23.5182, -3.0181) knots 0 0 0 1 2 2 2
  spline S223 degree 2 poles (-23.5182, -3.0181) (-23.4626, -3.4519) (-23.5773, -4.1263) (-23.7207, -4.3563) knots 0 0 0 1 2 2 2
  spline S224 degree 2 poles (-23.7207, -4.3563) (-23.8645, -4.5829) (-24.3012, -4.8364) (-24.5581, -4.8693) knots 0 0 0 1 2 2 2
  spline S225 degree 2 poles (-24.5581, -4.8693) (-24.926, -4.9164) (-25.4674, -4.573) (-25.6799, -4.2087) knots 0 0 0 1 2 2 2
  line L266 (-25.6799, -4.2087) -> (-25.6972, -4.2109)
  spline S226 degree 2 poles (-25.6972, -4.2109) (-25.8327, -4.6128) (-26.3186, -4.9784) (-26.6414, -5.0198) knots 0 0 0 1 2 2 2
  spline S227 degree 2 poles (-26.6414, -5.0198) (-26.8774, -5.05) (-27.3171, -4.8947) (-27.5064, -4.7108) knots 0 0 0 1 2 2 2
  spline S228 degree 2 poles (-27.5064, -4.7108) (-27.688, -4.533) (-27.9523, -3.9565) (-28.0003, -3.5817) knots 0 0 0 1 2 2 2
  spline S229 degree 2 poles (-28.0003, -3.5817) (-28.051, -3.186) (-27.9565, -2.5742) (-27.8422, -2.3655) knots 0 0 0 1 2 2 2
  spline S230 degree 2 poles (-27.8422, -2.3655) (-27.7282, -2.1533) (-27.3523, -1.8935) (-27.1197, -1.8637) knots 0 0 0 1 2 2 2
  spline S231 degree 2 poles (-27.1197, -1.8637) (-26.8143, -1.8246) (-26.2796, -2.1159) (-26.0628, -2.4586) knots 0 0 0 1 2 2 2
  line L267 (-26.0628, -2.4586) -> (-26.0489, -2.4568)
  spline S232 degree 2 poles (-26.0489, -2.4568) (-25.9301, -2.0076) (-25.4194, -1.533) (-25.0272, -1.4828) knots 0 0 0 1 2 2 2
  spline S233 degree 2 poles (-24.846, -2.5391) (-25.0577, -2.5662) (-25.2567, -2.7751) (-25.3617, -3.0849) knots 0 0 0 1 2 2 2
  spline S234 degree 2 poles (-25.3617, -3.0849) (-25.3892, -3.1731) (-25.4702, -3.5045) (-25.5067, -3.6326) knots 0 0 0 1 2 2 2
  spline S235 degree 2 poles (-25.5067, -3.6326) (-25.3814, -3.7295) (-25.0255, -3.8638) (-24.8277, -3.8385) knots 0 0 0 1 2 2 2
  spline S236 degree 2 poles (-24.8277, -3.8385) (-24.5292, -3.8002) (-24.2206, -3.3726) (-24.2602, -3.0637) knots 0 0 0 1 2 2 2
  spline S237 degree 2 poles (-24.2602, -3.0637) (-24.2713, -2.977) (-24.3544, -2.7689) (-24.4206, -2.6927) knots 0 0 0 1 2 2 2
  spline S238 degree 2 poles (-24.4206, -2.6927) (-24.4986, -2.6074) (-24.6933, -2.5195) (-24.846, -2.5391) knots 0 0 0 1 2 2 2
  spline S239 degree 2 poles (-26.861, -2.8924) (-27.0796, -2.9204) (-27.303, -3.2419) (-27.2715, -3.4883) knots 0 0 0 1 2 2 2
  spline S240 degree 2 poles (-27.2715, -3.4883) (-27.2412, -3.7243) (-26.9683, -3.9822) (-26.7948, -3.9599) knots 0 0 0 1 2 2 2
  spline S241 degree 2 poles (-26.7948, -3.9599) (-26.6247, -3.9381) (-26.4352, -3.7375) (-26.372, -3.5424) knots 0 0 0 1 2 2 2
  spline S242 degree 2 poles (-26.372, -3.5424) (-26.3406, -3.4572) (-26.2823, -3.224) (-26.2364, -3.0311) knots 0 0 0 1 2 2 2
  spline S243 degree 2 poles (-26.2364, -3.0311) (-26.3964, -2.9387) (-26.6839, -2.8697) (-26.861, -2.8924) knots 0 0 0 1 2 2 2
  dimension "d145" = 47.625
  constraints: 1 centre point, 1 coincident, 1 other
  measures "d145" diameter of A0
extrude "Extrusion19" cut sketch "Sketch26" against normal blind 1.905
sketch "Sketch27" plane through (0, 72.39, 0) normal (0, 1, 0) x (1, 0, 0)
  line L0 (-3.9595, 6.858) -> (3.9595, 6.858)
  line L1 (3.9595, 6.858) -> (7.9189, 0)
  line L2 (7.9189, 0) -> (3.9595, -6.858)
  line L3 (3.9595, -6.858) -> (-3.9595, -6.858)
  line L4 (-3.9595, -6.858) -> (-7.9189, 0)
  line L5 (-7.9189, 0) -> (-3.9595, 6.858)
  point P0 (0, 0)
  point P1 (0, 0)
  dimension "d153" = 13.716
  constraints: 12 end point, 1 coincident, 1 horizontal, 13 other
  measures "d153" distance between parallel lines of L0 L3
extrude "Extrusion20" cut sketch "Sketch27" against normal through all
equation "\"d103\" = hexDiameter"
equation "\"d110\" = centerLineForSpool"
equation "\"d111\" = centerLineForSpool"
equation "\"d112\" = holeForString"
equation "\"d121\" = centerLineForSpool"
equation "\"d122\" = holeForString"
equation "\"d125\" = knotHoleDiameter"
equation "\"d127\" = holeForString"
equation "\"d128\" = centerLineForSpool"
equation "\"d129\" = knotHoleDiameter"
equation "\"d130\" = knotHoleDepth"
equation "\"d85\" = spoolExteriorRadius"
equation "\"d86\" = spoolOverallHeight"
equation "\"d88\" = d85"
equation "\"d89\" = 0.5 * spoolOverallHeight"
equation "\"centerLineForSpool\" = 0.25 * spoolOverallHeight"
equation "\"holeForString\" = stringDiameter + clearanceForString"
equation "\"stringDiameter\" = 3.048"
equation "\"clearanceForString\" = 2.032"
equation "\"hexShaftDiameter\" = 12.7"
equation "\"clearanceForHexShaft\" = 1.016"
equation "\"hexDiameter\" = hexShaftDiameter + clearanceForHexShaft"
equation "\"spoolInteriorDiameter\" = 38.1"
equation "\"spoolInteriroRadius\" = 0.5 * spoolInteriorDiameter"
equation "\"spoolExteriorDiameter\" = 63.5"
equation "\"spoolExteriorRadius\" = 0.5 * spoolExteriorDiameter"
equation "\"hexHoleChamfer\" = 1.5875"
equation "\"stringHoleCenterFromHexShaft\" = 0.5 * hexDiameter + 0.5 * holeForString"
equation "\"textCircleDiameter\" = 0.75 * spoolExteriorDiameter"
equation "\"textHeight\" = 4.572"
equation "\"textDepth\" = 1.27"
equation "\"spoolOverallHeight\" = 69.85"
equation "\"d114\" = -spoolInteriroRadius"
equation "\"knotHoleDiameter\" = 9.525"
equation "\"d126\" = spoolInteriroRadius"
equation "\"metalWasherID\" = 26.67"
equation "\"metalWasherThickness\" = 2.54"
equation "\"spacerOD\" = 24.13"
equation "\"spacerThickness\" = 2.54"
equation "\"knotHoleDepth\" = 11.1125"
body "Solid3"
